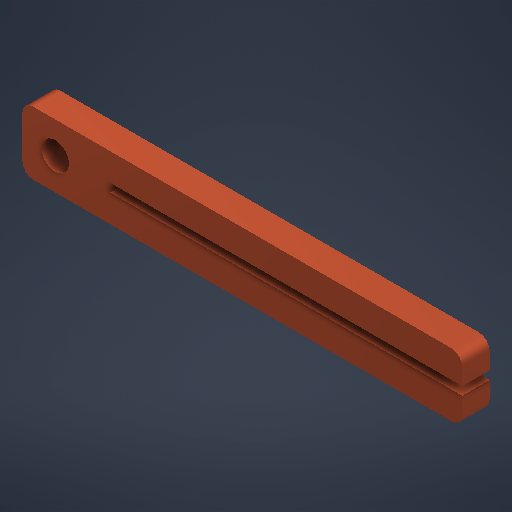
# Autodesk Inventor part: Bush_phase_mono
Saved by Autodesk Inventor 2026.2 (Build 302298000, 298)
## iProperties
Created: 2026-01-22
Part Number: Bush_phase_mono
Material: Медь
Document SubType Name: Modeling
Designer: EV-TECH
Density: 8.94 g/cm^3
Appearance: Медь — сатинированная
Author: EV-TECH
Autodesk Inventor part; units mm, degrees
ref_plane "YZ Plane" through (0, 0, 0) normal (1, 0, 0) x (0, 1, 0)
ref_plane "XZ Plane" through (0, 0, 0) normal (0, 1, 0) x (-1, 0, 0)
ref_plane "XY Plane" through (0, 0, 0) normal (0, 0, 1) x (1, 0, 0)
sketch "Эскиз1" plane through (0, 0, 0) normal (0, 1, 0) x (-1, 0, 0)
  point P0 (0, 0)
sketch "Эскиз2" plane through (0, 0, 0) normal (0, 0, 1) x (1, 0, 0)
  line L0 (0, 0) -> (80, 0)
  line L1 (80, 0) -> (80, 5)
  line L2 (80, 5) -> (0, 5)
  line L3 (0, 5) -> (0, 0)
  line L4 (0, 5) -> (16, 5)
  line L5 (16, 5) -> (16, 6.5)
  line L6 (16, 6.5) -> (0, 6.5)
  line L7 (0, 6.5) -> (0, 5)
  line L8 (0, 6.5) -> (80, 6.5)
  line L9 (80, 6.5) -> (80, 11.5)
  line L10 (80, 11.5) -> (0, 11.5)
  line L11 (0, 11.5) -> (0, 6.5)
  dimension "d0" = 5
  dimension "d1" = 80
  dimension "d2" = 16
  dimension "d3" = 1.5
  dimension "d4" = 80
  dimension "d5" = 5
  constraints: 24 end point, 6 parallel, 3 horizontal, 3 perpendicular
  measures "d0" distance of L0.end L1.end
  measures "d1" distance of L1.end L2.end
  measures "d2" distance of L5.end L6.end
  measures "d3" distance of L4.end L5.end
  measures "d4" distance of L9.end L10.end
  measures "d5" distance of L8.end L9.end
extrude "Выдавливание1" add sketch "Эскиз2" along normal blind 5
fillet "Сопряжение1" radius 2 4 edges at (0, 0, 2.5) (0, 11.5, 2.5) (80, 0, 2.5) (80, 11.5, 2.5)
sketch "Эскиз3" plane through (0, 0, 0) normal (0, 0, -1) x (-1, 0, 0)
  circle A0 centre (-6, 5.75) radius 2.5
  line L0 (-16, 5) -> (-16, 6.5) projected
  line L1 (-16, 5.75) -> (-16, 5)
  point P0 (0, 0)
  dimension "d9" = 5
  constraints: 2 end point, 1 centre point
  measures "d9" diameter of A0
extrude "Выдавливание2" cut sketch "Эскиз3" against normal blind 13.75
